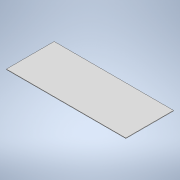
# Autodesk Inventor part: 2.5ftX12in
Saved by Autodesk Inventor 2020 (Build 240168000, 168)
## iProperties
Created: 2021-11-12
Part Number: 2.5ftX12in
Material: Generic
Document SubType Name: Sheet Metal
Designer: 17185
Density: 1 g/cm^3
Sheet Metal Rule: Default
Appearance: Default
Author: 17185
Autodesk Inventor part; units mm, degrees
ref_plane "YZ Plane" through (0, 0, 0) normal (1, 0, 0) x (0, 1, 0)
ref_plane "XZ Plane" through (0, 0, 0) normal (0, 1, 0) x (-1, 0, 0)
ref_plane "XY Plane" through (0, 0, 0) normal (0, 0, 1) x (1, 0, 0)
sketch "Sketch1" plane through (0, 0, 0) normal (0, 1, 0) x (-1, 0, 0)
  line L0 (381, 152.4) -> (-381, 152.4)
  line L1 (-381, 152.4) -> (-381, -152.4)
  line L2 (-381, -152.4) -> (381, -152.4)
  line L3 (381, -152.4) -> (381, 152.4)
  line L4 (381, 152.4) -> (-381, -152.4) construction
  line L5 (-381, 152.4) -> (381, -152.4) construction
  point P0 (0, 0)
  dimension "d0" = 304.8
  dimension "d1" = 762
  measures "d0" distance of L0.end L1.end
  measures "d1" distance of L1.end L2.end
extrude "Plate1" add sketch "Sketch1" along normal blind 3.048
equation "\"d2\" = Thickness"
equation "\"BendRadius\" = Thickness"
equation "\"BendReliefWidth\" = Thickness"
equation "\"BendReliefDepth\" = 0.5 * Thickness"
equation "\"CornerReliefSize\" = 4 * Thickness"
equation "\"MinimumRemnant\" = 2 * Thickness"
equation "\"TransitionRadius\" = BendRadius"
equation "\"JacobiRadiusSize\" = BendRadius"
equation "\"GapSize\" = Thickness"
equation "\"Thickness\" = 3.048"
body "Solid1"
